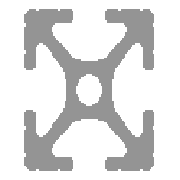
# Autodesk Inventor part: 8020 Profile
Saved by Autodesk Inventor 2012 (Build 160160000, 160)
## iProperties
Created: 2011-08-07
Part Number: 8020 Profile
Material: Default
Document SubType Name: Modeling
Designer: Ian Walters
Density: 1 g/cm^3
Categories: <MemberInstance><Categories><Category DisplayName="Structural Shapes" InternalName="089c4875-fa83-4c05-b084-43b9cc11f5ed" Mnemonic="GRDR"><CategoryParameter DisplayName="Custom Base Point" InternalName="4f1d1b73-316d-484b-a3df-9cbabb16eb77" Mnemonic="shpBasePoint"/><CategoryParameter DisplayName="FG Authored" InternalName="9c666724-f362-4ea7-ac62-f6a007de5c69" Mnemonic="shpFGAuto"/><CategoryParameter DisplayName="Legacy Member ID" InternalName="340afe4f-75d7-48d3-ab7d-943f3c3da468" Mnemonic="LegacyMemberID"/><CategoryParameter DisplayName="Base Length" InternalName="42e34263-8f20-4d0e-ad48-bf1385b87c24" Mnemonic="shplen"/><CategoryParameter DisplayName="Distance of the Center of Gravity X-X" InternalName="26c9bdb8-9c79-4b4f-a92e-8e197583c9c4" Mnemonic="grcendistX"/><CategoryParameter DisplayName="Distance of the Center of Gravity Y-Y" InternalName="bcc4fb17-7af4-436a-8f8c-d0aa3b0248c5" Mnemonic="grcendistY"/><CategoryParameter DisplayName="Torsional Rigidity Modulus" InternalName="26c1ec35-5026-4c63-ad0a-751cf684a536" Mnemonic="torrigmod"/><CategoryParameter DisplayName="Torsional Section Modulus" InternalName="7c55a8dc-8844-49f9-a867-cc677b30ec9a" Mnemonic="torsecmod"/><CategoryParameter DisplayName="Coefficient of Shear Displacement" InternalName="de4c90c6-aaa8-468f-a335-6737b311b5d3" Mnemonic="shdispc"/><CategoryParameter DisplayName="Section Area" InternalName="1ff91680-64b0-4202-b9a3-7fd3f94bba3b" Mnemonic="secarea"/><CategoryParameter DisplayName="Moment of Inertia (x)" InternalName="4cd780bc-73d7-43ac-917a-579e5cbd684d" Mnemonic="inermomx"/><CategoryParameter DisplayName="Moment of Inertia (y)" InternalName="4b9f58ea-bced-460e-81ea-3d29ca5a49e3" Mnemonic="inermomy"/><CategoryParameter DisplayName="Section Module (x)" InternalName="72cfad18-cf51-4ed4-aaa7-c6b224f8419f" Mnemonic="secmodx"/><CategoryParameter DisplayName="Section Module (y)" InternalName="59eaa5e9-d227-48dc-b6c1-6920f96e0f95" Mnemonic="secmody"/><CategoryParameter DisplayName="Radius of Gyration (x)" InternalName="25778675-03e9-40c1-b6a8-4a9ed693320d" Mnemonic="gyrradx"/><CategoryParameter DisplayName="Radius of Gyration (y)" InternalName="bfa18ebe-1636-4dbe-8d42-b263e0b73184" Mnemonic="gyrrady"/><CategoryParameter DisplayName="Shape Thickness" InternalName="d109cf76-8eb4-42fc-9800-4409734adc67" Mnemonic="shpthick"/><CategoryParameter DisplayName="Second Shape Thickness" InternalName="9251a8e1-85fd-4e47-af99-afdb762317d9" Mnemonic="shpthick2"/><CategoryParameter DisplayName="Shape Width" InternalName="7c717d54-a18f-4666-b4d4-573cce22c62c" Mnemonic="shpwdth"/><CategoryParameter DisplayName="Shape Height" InternalName="50274e7d-5ac0-4796-92cb-c59e54983c67" Mnemonic="shpheig"/><CategoryParameter DisplayName="Mass per Length Unit" InternalName="0bb95a10-148f-4027-a459-38d7b056702a" Mnemonic="shpmass"/><CategoryParameter DisplayName="Section Designation" InternalName="5a64d034-428d-49c8-ba32-7619764de20f" Mnemonic="shpdes"/><Category DisplayName="Square/Rectangular Tubes" InternalName="afc8e2d8-05d6-4609-8807-f98a9b7d2ed0" Mnemonic="SQRSHP"><CategoryParameter DisplayName="Moment of Inertia (x)" InternalName="8c4637b6-6b69-4878-9d5d-26a32185d655" Mnemonic="inermomx"/><CategoryParameter DisplayName="Moment of Inertia (y)" InternalName="55ec8510-8276-4c45-8f10-594e0fee7eb3" Mnemonic="inermomy"/><CategoryParameter DisplayName="Section Module (x)" InternalName="50d965a6-04bf-46b9-8ace-861858d348e6" Mnemonic="secmodx"/><CategoryParameter DisplayName="Section Module (y)" InternalName="5106aeac-54a2-4159-a9af-8933dd39dba2" Mnemonic="secmody"/><CategoryParameter DisplayName="Section Area" InternalName="2f7f79dd-983c-4263-802a-5b6a1495fdc5" Mnemonic="secarea"/><CategoryParameter DisplayName="Radius of Gyration (x)" InternalName="56c89926-a299-4389-a862-ac94c9691272" Mnemonic="gyrradx"/><CategoryParameter DisplayName="Radius of Gyration (y)" InternalName="fa48a7f5-f030-40f9-a60b-de8a845b7104" Mnemonic="gyrrady"/><CategoryParameter DisplayName="Shape Width" InternalName="8c8a1782-5e80-4d77-858b-304b1c0ad1fd" Mnemonic="shpwdth"/><CategoryParameter DisplayName="Shape Thickness" InternalName="52712fc5-f4ee-4eda-b3f2-6fce82c26419" Mnemonic="shpthick"/><CategoryParameter DisplayName="Radius" InternalName="5d8d062c-e28e-41c1-98da-8e5fee36da1a" Mnemonic="shprad"/></Category></Category></Categories><FamilyTemplate Id="8020 Profile"><FamilyTemplateParameters><FamilyTemplateParameter ObjectType="kModelParameterObject" ValueType="xs:double" Id="12" ObjectReferenceKey="length"/></FamilyTemplateParameters></FamilyTemplate><CategoryParameterMap><ParamToTemplateMap><ParamToTemplate CategoryParameter="//CategoryParameter[@InternalName='42e34263-8f20-4d0e-ad48-bf1385b87c24']" TemplateParameter="12"/><ParamToTemplate CategoryParameter="//CategoryParameter[@InternalName='9c666724-f362-4ea7-ac62-f6a007de5c69']" ConstantValue="1"/><ParamToTemplate CategoryParameter="//CategoryParameter[@InternalName='4f1d1b73-316d-484b-a3df-9cbabb16eb77']" ConstantValue="1"/></ParamToTemplateMap></CategoryParameterMap></MemberInstance>
G_L: 2.000 in
Author: Ian Walters
Autodesk Inventor part; units mm, degrees
ref_plane "YZ Plane" through (0, 0, 0) normal (1, 0, 0) x (0, 1, 0)
ref_plane "Start Plane" through (0, 0, 0) normal (0, 0, 1) x (1, 0, 0)
ref_plane "End Plane" through (0, 0, 50.8) normal (0, 0, 1) x (1, 0, 0)
sketch "Sketch2" plane through (0, 0, 0) normal (0, 0, 1) x (1, 0, 0)
  line L0 (-11.651, 3.2385) -> (-11.5392, 3.2385)
  line L1 (-10.4902, 4.2875) -> (-10.4902, 6.4472)
  line L2 (-8.7363, 7.1737) -> (-5.4384, 3.8759)
  line L3 (-4.5085, 1.6308) -> (-4.5085, 0)
  line L4 (-3.2385, 11.651) -> (-3.2385, 11.5392)
  line L5 (-4.2875, 10.4902) -> (-6.4472, 10.4902)
  line L6 (-7.1737, 8.7363) -> (-3.8759, 5.4384)
  line L7 (-1.6308, 4.5085) -> (0, 4.5085)
  line L8 (-12.7, 12.7) -> (0, 0) construction
  line L9 (0, 12.7) -> (0, 0) construction
  line L10 (0, 0) -> (-12.7, 0) construction
  arc A0 (-10.5918, 12.7) -> (-12.7, 10.5918) centre (-10.5918, 10.5918) ccw
  arc A1 (-12.7, 4.2875) -> (-11.651, 3.2385) centre (-11.651, 4.2875) ccw
  arc A2 (-11.5392, 3.2385) -> (-10.4902, 4.2875) centre (-11.5392, 4.2875) ccw
  arc A3 (-4.2875, 10.4902) -> (-3.2385, 11.5392) centre (-4.2875, 11.5392) ccw
  arc A4 (-3.2385, 11.651) -> (-4.2875, 12.7) centre (-4.2875, 11.651) ccw
  arc A5 (-4.5085, 1.6308) -> (-5.4384, 3.8759) centre (-7.6835, 1.6308) ccw
  arc A6 (-3.8759, 5.4384) -> (-1.6308, 4.5085) centre (-1.6308, 7.6835) ccw
  arc A7 (-8.7363, 7.1737) -> (-10.4902, 6.4472) centre (-9.4628, 6.4472) ccw
  arc A8 (-6.4472, 10.4902) -> (-7.1737, 8.7363) centre (-6.4472, 9.4628) ccw
  arc A9 (0, 2.6035) -> (-2.6035, 0) centre (0, 0) ccw
  arc A10 (-10.5664, 12.7) -> (-9.5504, 12.7) centre (-10.0584, 12.7) ccw
  arc A11 (-6.3331, 12.7) -> (-5.3171, 12.7) centre (-5.8251, 12.7) ccw
  arc A12 (-12.7, 9.5504) -> (-12.7, 10.5664) centre (-12.7, 10.0584) ccw
  arc A13 (-12.7, 5.3171) -> (-12.7, 6.3331) centre (-12.7, 5.8251) ccw
  line L11 (-4.2875, 12.7) -> (-5.3171, 12.7)
  line L12 (-6.3331, 12.7) -> (-9.5504, 12.7)
  line L13 (-10.5664, 12.7) -> (-10.5918, 12.7)
  line L14 (-12.7, 10.5918) -> (-12.7, 10.5664)
  line L15 (-12.7, 9.5504) -> (-12.7, 6.3331)
  line L16 (-12.7, 5.3171) -> (-12.7, 4.2875)
  line L17 (11.651, 3.2385) -> (11.5392, 3.2385)
  line L18 (10.4902, 4.2875) -> (10.4902, 6.4472)
  line L19 (8.7363, 7.1737) -> (5.4384, 3.8759)
  line L20 (4.5085, 1.6308) -> (4.5085, 0)
  line L21 (3.2385, 11.651) -> (3.2385, 11.5392)
  line L22 (4.2875, 10.4902) -> (6.4472, 10.4902)
  line L23 (7.1737, 8.7363) -> (3.8759, 5.4384)
  line L24 (1.6308, 4.5085) -> (0, 4.5085)
  arc A14 (12.7, 10.5918) -> (10.5918, 12.7) centre (10.5918, 10.5918) ccw
  arc A15 (11.651, 3.2385) -> (12.7, 4.2875) centre (11.651, 4.2875) ccw
  arc A16 (10.4902, 4.2875) -> (11.5392, 3.2385) centre (11.5392, 4.2875) ccw
  arc A17 (3.2385, 11.5392) -> (4.2875, 10.4902) centre (4.2875, 11.5392) ccw
  arc A18 (4.2875, 12.7) -> (3.2385, 11.651) centre (4.2875, 11.651) ccw
  arc A19 (5.4384, 3.8759) -> (4.5085, 1.6308) centre (7.6835, 1.6308) ccw
  arc A20 (1.6308, 4.5085) -> (3.8759, 5.4384) centre (1.6308, 7.6835) ccw
  arc A21 (10.4902, 6.4472) -> (8.7363, 7.1737) centre (9.4628, 6.4472) ccw
  arc A22 (7.1737, 8.7363) -> (6.4472, 10.4902) centre (6.4472, 9.4628) ccw
  arc A23 (2.6035, 0) -> (0, 2.6035) centre (0, 0) ccw
  arc A24 (9.5504, 12.7) -> (10.5664, 12.7) centre (10.0584, 12.7) ccw
  arc A25 (5.3171, 12.7) -> (6.3331, 12.7) centre (5.8251, 12.7) ccw
  arc A26 (12.7, 10.5664) -> (12.7, 9.5504) centre (12.7, 10.0584) ccw
  arc A27 (12.7, 6.3331) -> (12.7, 5.3171) centre (12.7, 5.8251) ccw
  line L25 (4.2875, 12.7) -> (5.3171, 12.7)
  line L26 (6.3331, 12.7) -> (9.5504, 12.7)
  line L27 (10.5664, 12.7) -> (10.5918, 12.7)
  line L28 (12.7, 10.5918) -> (12.7, 10.5664)
  line L29 (12.7, 9.5504) -> (12.7, 6.3331)
  line L30 (12.7, 5.3171) -> (12.7, 4.2875)
  line L31 (-11.651, -3.2385) -> (-11.5392, -3.2385)
  line L32 (-10.4902, -4.2875) -> (-10.4902, -6.4472)
  line L33 (-8.7363, -7.1737) -> (-5.4384, -3.8759)
  line L34 (-3.2385, -11.651) -> (-3.2385, -11.5392)
  line L35 (-4.2875, -10.4902) -> (-6.4472, -10.4902)
  line L36 (-7.1737, -8.7363) -> (-3.8759, -5.4384)
  line L37 (-1.6308, -4.5085) -> (0, -4.5085)
  arc A28 (-12.7, -10.5918) -> (-10.5918, -12.7) centre (-10.5918, -10.5918) ccw
  arc A29 (-11.651, -3.2385) -> (-12.7, -4.2875) centre (-11.651, -4.2875) ccw
  arc A30 (-10.4902, -4.2875) -> (-11.5392, -3.2385) centre (-11.5392, -4.2875) ccw
  arc A31 (-3.2385, -11.5392) -> (-4.2875, -10.4902) centre (-4.2875, -11.5392) ccw
  arc A32 (-4.2875, -12.7) -> (-3.2385, -11.651) centre (-4.2875, -11.651) ccw
  arc A33 (-5.4384, -3.8759) -> (-4.5085, -1.6308) centre (-7.6835, -1.6308) ccw
  arc A34 (-1.6308, -4.5085) -> (-3.8759, -5.4384) centre (-1.6308, -7.6835) ccw
  arc A35 (-10.4902, -6.4472) -> (-8.7363, -7.1737) centre (-9.4628, -6.4472) ccw
  arc A36 (-7.1737, -8.7363) -> (-6.4472, -10.4902) centre (-6.4472, -9.4628) ccw
  arc A37 (-9.5504, -12.7) -> (-10.5664, -12.7) centre (-10.0584, -12.7) ccw
  arc A38 (-5.3171, -12.7) -> (-6.3331, -12.7) centre (-5.8251, -12.7) ccw
  arc A39 (-12.7, -10.5664) -> (-12.7, -9.5504) centre (-12.7, -10.0584) ccw
  arc A40 (-12.7, -6.3331) -> (-12.7, -5.3171) centre (-12.7, -5.8251) ccw
  line L38 (-4.2875, -12.7) -> (-5.3171, -12.7)
  line L39 (-6.3331, -12.7) -> (-9.5504, -12.7)
  line L40 (-10.5664, -12.7) -> (-10.5918, -12.7)
  line L41 (-12.7, -10.5918) -> (-12.7, -10.5664)
  line L42 (-12.7, -9.5504) -> (-12.7, -6.3331)
  line L43 (-12.7, -5.3171) -> (-12.7, -4.2875)
  line L44 (10.4902, -4.2875) -> (10.4902, -6.4472)
  arc A41 (4.5085, -1.6308) -> (5.4384, -3.8759) centre (7.6835, -1.6308) ccw
  line L45 (8.7363, -7.1737) -> (5.4384, -3.8759)
  line L46 (7.1737, -8.7363) -> (3.8759, -5.4384)
  arc A42 (3.8759, -5.4384) -> (1.6308, -4.5085) centre (1.6308, -7.6835) ccw
  line L47 (11.651, -3.2385) -> (11.5392, -3.2385)
  line L48 (4.2875, -10.4902) -> (6.4472, -10.4902)
  line L49 (4.2875, -12.7) -> (5.3171, -12.7)
  arc A43 (3.2385, -11.651) -> (4.2875, -12.7) centre (4.2875, -11.651) ccw
  line L50 (3.2385, -11.651) -> (3.2385, -11.5392)
  arc A44 (4.2875, -10.4902) -> (3.2385, -11.5392) centre (4.2875, -11.5392) ccw
  arc A45 (6.4472, -10.4902) -> (7.1737, -8.7363) centre (6.4472, -9.4628) ccw
  line L51 (6.3331, -12.7) -> (9.5504, -12.7)
  arc A46 (10.5664, -12.7) -> (9.5504, -12.7) centre (10.0584, -12.7) ccw
  line L52 (10.5664, -12.7) -> (10.5918, -12.7)
  arc A47 (10.5918, -12.7) -> (12.7, -10.5918) centre (10.5918, -10.5918) ccw
  arc A48 (6.3331, -12.7) -> (5.3171, -12.7) centre (5.8251, -12.7) ccw
  arc A49 (12.7, -4.2875) -> (11.651, -3.2385) centre (11.651, -4.2875) ccw
  arc A50 (11.5392, -3.2385) -> (10.4902, -4.2875) centre (11.5392, -4.2875) ccw
  arc A51 (8.7363, -7.1737) -> (10.4902, -6.4472) centre (9.4628, -6.4472) ccw
  line L53 (12.7, -10.5918) -> (12.7, -10.5664)
  arc A52 (12.7, -9.5504) -> (12.7, -10.5664) centre (12.7, -10.0584) ccw
  arc A53 (12.7, -5.3171) -> (12.7, -6.3331) centre (12.7, -5.8251) ccw
  line L54 (12.7, -5.3171) -> (12.7, -4.2875)
  line L55 (12.7, -9.5504) -> (12.7, -6.3331)
  line L56 (1.6308, -4.5085) -> (0, -4.5085)
  line L57 (-4.5085, -1.6308) -> (-4.5085, 0)
  arc A54 (-2.6035, 0) -> (0, -2.6035) centre (0, 0) ccw
  arc A55 (0, -2.6035) -> (2.6035, 0) centre (0, 0) ccw
  line L58 (4.5085, -1.6308) -> (4.5085, 0)
  line L59 (-12.7, 12.7) -> (12.7, 12.7)
  line L60 (12.7, 12.7) -> (12.7, -12.7)
  line L61 (12.7, -12.7) -> (-12.7, -12.7)
  line L62 (-12.7, -12.7) -> (-12.7, 12.7)
  point P0 (-3.2385, 12.7)
  point P1 (-12.7, 3.2385)
  point P2 (-3.2385, 10.4902)
  point P3 (3.2385, 12.7)
  point P4 (12.7, 3.2385)
  point P5 (3.2385, 10.4902)
  point P6 (-3.2385, -12.7)
  point P7 (-12.7, -3.2385)
  point P8 (-3.2385, -10.4902)
  point P9 (0, -12.7)
  point P10 (12.7, -3.2385)
  point P11 (3.2385, -12.7)
  point P12 (3.2385, -10.4902)
  point P13 (0, 12.7)
  dimension "d1" = 2.2098
  dimension "d2" = 3.2385
  dimension "d3" = 2.2098
  dimension "d4" = 4.5085
  dimension "d5" = 2.1082
  dimension "d6" = 1.049
  dimension "d7" = 3.175
  dimension "d8" = 1.0274
  dimension "d9" = 2.6035
  dimension "d10" = 2.5866
  dimension "d11" = 0.508
  dimension "d12" = 2.5866
  dimension "d13" = 3.2385
  dimension "d14" = 12.7
  dimension "d15" = 2.6416
  dimension "d16" = 2.2098
  dimension "d17" = 2.6416
  constraints: 135 symmetric about line, 126 end point, 112 point on circle, 56 centre point, 34 point on line, 26 tangent, 17 perpendicular, 15 parallel, 8 equal radius, 5 horizontal alignment, 5 vertical alignment, 4 horizontal, 2 midpoint, 1 coincident, 42 other
  measures "d1" distance of point (-3.239, 12.7) point (-3.239, 10.49)
  measures "d2" distance between parallel lines of L9 L4
  measures "d3" distance between parallel lines of L6 L2
  measures "d4" distance between parallel lines of L10 L7
  measures "d5" radius of A0
  measures "d6" radius of A1
  measures "d7" radius of A5
  measures "d8" radius of A7
  measures "d9" radius of A9
  measures "d10" distance from line of L4 A11.centre
  measures "d11" radius of A10
  measures "d12" distance from line of L0 A13.centre
  measures "d13" distance between parallel lines of L10 L0
  measures "d14" distance of L8.end L10.end
  measures "d15" distance from line of L14 A10.centre
  measures "d16" distance between parallel lines of L1 L16
  measures "d17" distance from line of L12 A12.centre
extrude "Body" add sketch "Sketch2" along normal up to surface (50.8 mm away) from surface at 0 contours A1 L16 A13 L15 A12 L14 A0 L13 A10 L12 A11 L11 A4 L4 A3 L5 A8 L6 A6 L7 L24 A20 L23 A22 L22 A17 L21 A18 L25 A25 L26 A24 L27 A14 L28 A26 L29 A27 L30 A15 L17 A16 L18 A21 L19 A19 L20 L58 A41 L45 A51 L44 A50 L47 A49 L54 A53 L55 A52 L53 A47 L52 A46 L51 A48 L49 A43 L50 A44 L48 A45 L46 A42 L56 L37 A34 L36 A36 L35 A31 L34 A32 L38 A38 L39 A37 L40 A28 L41 A39 L42 A40 L43 A29 L31 A30 L32 A35 L33 A33 L57 L3 A5 L2 A7 L1 A2 L0
sketch "Sketch9" plane through (0, 0, 0) normal (0, 0, 1) x (1, 0, 0)
  line L0 (0, 0) -> (10, 0)
ref_plane "Work Plane6" through (0, 0, 0) normal (0, -1, 0) x (1, 0, 0)
sketch "Sketch10" plane through (0, 0, 0) normal (0, -1, 0) x (1, 0, 0)
  line L0 (-17.78, 0) -> (17.78, 0)
  line L1 (-17.78, 50.8) -> (17.78, 50.8)
  dimension "d28" = 50.8
  measures "d28" distance between parallel lines of L0 L1
equation "\"d3\" = d1"
equation "\"d12\" = d10"
equation "\"d13\" = d2"
equation "\"G_OFFSET_START\" = 0"
equation "\"G_OFFSET_END\" = 0"
equation "\"G_L\" = 50.8"
body "Solid1"
